nixal_reprap4040_Xtensioner (Autodesk Fusion 360 design; units mm, degrees)
Autodesk Fusion 360 part; units mm, degrees
sketch "Sketch1" plane through (0, 0, 0) normal (0, 1, 0) x (1, 0, 0)
  line L0 (0, 0) -> (10, 0)
  line L1 (10, 1.5) -> (10, 8.5)
  line L2 (10, 10) -> (0, 10)
  line L3 (0, 10) -> (0, 0)
  line L4 (10, 10) -> (35, 10)
  line L5 (35, 10) -> (35, 8.5)
  line L6 (35, 8.5) -> (10, 8.5)
  line L7 (10, 0) -> (35, 0)
  line L8 (35, 0) -> (35, 1.5)
  line L9 (35, 1.5) -> (10, 1.5)
  line L10 (6.5, 7.65) -> (3.5, 7.65)
  line L11 (3.5, 7.65) -> (3.5, 2.35)
  line L12 (3.5, 2.35) -> (6.5, 2.35)
  line L13 (6.5, 2.35) -> (6.5, 7.65)
  line L14 (6.5, 7.65) -> (3.5, 2.35) construction
  line L15 (3.5, 7.65) -> (6.5, 2.35) construction
  dimension "d1" = 10
  dimension "d2" = 10
  dimension "d3" = 5.3
  dimension "d4" = 3
  constraint horizontal L0
  constraint vertical L1
  constraint horizontal L2
  constraint vertical L3
  constraint coincident L0.start L3.end
  constraint perpendicular L1 L4
  constraint perpendicular L4 L5
  constraint perpendicular L1 L6
  constraint perpendicular L1 L7
  constraint perpendicular L7 L8
  constraint perpendicular L1 L9
  constraint perpendicular L10 L11
  constraint parallel L10 L12
  constraint parallel L11 L13
  constraint horizontal L10
  constraint coincident L14 L0.start
  constraint coincident L15 L0.start
  measures "d2" distance of L0.start
  measures "d3" distance of L0.start
extrude "Extrude1" add sketch "Sketch1" along normal blind 10 makes body 1
sketch "Sketch2" plane through (0, 0, 0) normal (0, 0, 1) x (1, 0, 0)
  line L0 (0, 0) -> (35, 0)
  line L1 (35, 0) -> (35, 10)
  line L2 (35, 10) -> (0, 10)
  line L3 (0, 10) -> (0, 0)
  circle A0 centre (30, 5) radius 1.5
  circle A1 centre (30, 5) radius 4
  dimension "d7" = 3
  dimension "d8" = 8
  constraint concentric A0 A1
  measures "d7" diameter of A0
  measures "d8" diameter of A1
extrude "Extrude2" cut sketch "Sketch2" against normal blind 21 contours A0 bodies 1
extrude "Extrude3" add sketch "Sketch2" along normal blind -3 and the other way blind 1 separate body contours A1 makes body 2
fillet "Fillet1" radius 2 1 edges at (26.2707, 6.4465, -3) on bodies 2
extrude "Extrude4" add sketch "Sketch2" along normal blind -8.5 and the other way blind 7 separate body contours A1 makes body 3
fillet "Fillet2" radius 2.25 1 edges at (26.2707, 6.4465, -7) on bodies 3
sketch "Sketch3" plane through (0, 0, 0) normal (-1, 0, 0) x (0, 0, 1)
  line L0 (-10, 0) -> (0, 0)
  line L1 (0, 0) -> (0, 10)
  line L2 (0, 10) -> (-10, 10)
  line L3 (-10, 10) -> (-10, 0)
  circle A0 centre (-5, 5) radius 1.5
  dimension "d19" = 3
  measures "d19" diameter of A0
extrude "Extrude5" cut sketch "Sketch3" against normal blind 13 contours A0 bodies 1
